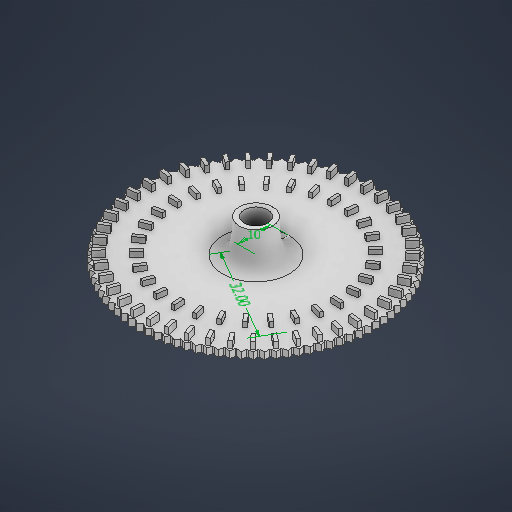
# Autodesk Inventor part: Диск v2
Saved by Autodesk Inventor 2026 (Build 300175000, 175)
## iProperties
Created: 2025-08-21
Part Number: Диск v2
Material: Типовые
Document SubType Name: Modeling
Designer: kvm13
Density: 1 g/cm^3
Appearance: По умолчанию
Author: kvm13
## iProperties of the stored document Диск v2_3DПЕЧАТЬ.ipt
Created: 2025-08-21
Part Number: Диск v2_3DПЕЧАТЬ
Material: Типовые
Document SubType Name: Modeling
Designer: kvm13
Density: 1 g/cm^3
Appearance: По умолчанию
Author: kvm13
Autodesk Inventor part; units mm, degrees
note: some values were not read from the file. Chosen so that the rebuilt part matches the saved one: pattern direction of "Круговой массив1".
ref_plane "YZ Plane" through (0, 0, 0) normal (1, 0, 0) x (0, 1, 0)
ref_plane "XZ Plane" through (0, 0, 0) normal (0, 1, 0) x (-1, 0, 0)
sketch "Эскиз1" plane through (0, 0, 0) normal (0, 1, 0) x (-1, 0, 0)
  circle A0 centre (0, 0) radius 35
  dimension "d0" = 70
  constraints: 1 centre point, 1 coincident
  measures "d0" diameter of A0
extrude "Выдавливание1" add sketch "Эскиз1" along normal blind 2
sketch "Эскиз2" plane through (0, 2, 0) normal (0, 1, 0) x (1, 0, 0)
  circle A0 centre (0, 0) radius 35 projected
  line L0 (0, 32) -> (-0.5, 32)
  line L1 (-0.5, 32) -> (-0.5, 34.9964)
  circle A1 centre (0, 0) radius 35 projected
  line L2 (0, 32) -> (0.5, 32)
  line L3 (0.5, 32) -> (0.5, 34.9964)
  dimension "d4" = 0.5
  constraints: 8 end point, 1 perpendicular, 3 other
  measures "d4" distance of L0.start L0.end
extrude "Выдавливание2" add sketch "Эскиз2" along normal blind 2 contours L3 L2 L0 L1 A0 picked at (-0.2222, 32.9999)
pattern_circular "Круговой массив1" count 45 over 360 about axis through (0, 0, 0) along (0, 1, 0) of "Выдавливание2"
sketch "Эскиз3" plane through (0, 2, 0) normal (0, 1, 0) x (1, 0, 0)
  line L0 (0.5, 32) -> (-0.5, 32) projected
  line L1 (-1.6712, 23.8986) -> (-1.1724, 23.9334)
  line L2 (-1.6712, 23.8986) -> (-2.1699, 23.8637)
  line L3 (-3.9584, 31.7582) -> (-4.3754, 34.7254) projected
  line L4 (-3.9584, 31.7582) -> (-0.5, 32)
  line L5 (-2.728, 31.8442) -> (-2.3792, 26.8564)
  line L6 (-2.3792, 26.8564) -> (-1.3816, 26.9261)
  line L7 (-1.3816, 26.9261) -> (-1.1724, 23.9334)
  line L8 (-2.3792, 26.8564) -> (-2.1699, 23.8637)
  point P0 (0, 0)
  point P1 (-1.4218, 23.916)
  dimension "d11" = 0.5
  dimension "d39" = 5
  dimension "d40" = 3
  constraints: 14 end point, 1 midpoint, 1 parallel
  measures "d11" distance of L1.start L1.end
  measures "d39" distance of L5.start L5.end
  measures "d40" distance of L5.end L2.end
extrude "Выдавливание3" add sketch "Эскиз3" along normal blind 1.5
sketch "Эскиз4" plane through (0, 0, 0) normal (0, -1, 0) x (1, 0, 0)
  line L0 (0, -35) -> (0, -36)
  line L1 (0, -36) -> (1.0147, -34.9853)
  line L2 (0, -36) -> (-1.0147, -34.9853)
  circle A0 centre (0, 0) radius 35
  dimension "d14" = 1
  dimension "d15" = 45
  constraints: 6 end point, 1 centre point, 1 coincident, 1 symmetric about line, 1 vertical
  measures "d14" distance of L0.start L0.end
  measures "d15" angle of L1 L0
extrude "Выдавливание4" add sketch "Эскиз4" against normal up to surface (2 mm away) contours A0 L1 L0 | L0 L2 A0
pattern_circular "Круговой массив2" count 90 over 360 about axis through (0, 0, 0) along (0, 1, 0) of "Выдавливание4"
pattern_circular "Круговой массив3" count 30 over 360 about axis through (0, 0, 0) along (0, 1, 0) of "Выдавливание3"
sketch "Эскиз5" plane through (0, 2, 0) normal (0, 1, 0) x (1, 0, 0)
  line L0 (0, 0) -> (0, 10)
  dimension "d24" = 10
  constraints: 2 end point, 1 vertical
  measures "d24" distance of L0.start L0.end
ref_plane "РабПлоскость1" through (0, 2, 0) normal (1, 0, 0) x (0, 0, -1)
sketch "Эскиз6" plane through (0, 2, 0) normal (1, 0, 0) x (0, 0, -1)
  line L0 (0, 0) -> (0, 10)
  line L1 (0, 0) -> (10, 0)
  line L2 (0, 0) -> (10, 0) projected
  line L3 (5, 10) -> (5, 2.9221) construction
  line L4 (5, 2.9221) -> (5.8227, 0) construction
  line L5 (5.8227, 0) -> (10, 0) construction
  spline S0 degree 3 poles (5, 10) (5, 2.9221) (5.8227, 0) (10, 0) knots 1 1 1 1 2 2 2 2
  line L6 (0, 10) -> (5, 10)
  point P0 (0, -2)
  dimension "d28" = 10
  dimension "d29" = 10
  dimension "d31" = 5
  constraints: 6 end point, 1 horizontal, 1 point on line, 1 vertical, 3 other
  measures "d28" distance of L0.start L1.end
  measures "d29" distance of L0.start L0.end
  measures "d31" distance of L0.end L3.start
revolve "Вращение1" add sketch "Эскиз6" angle 360 about axis through (0, 2, 0) along (0, 1, 0)
sketch "Эскиз7" plane through (0, 12, 0) normal (0, 1, 0) x (1, 0, 0)
  circle A0 centre (0, 0) radius 3.5
  point P0 (0, 0)
  dimension "d32" = 7
  constraints: 1 centre point, 1 coincident
  measures "d32" diameter of A0
extrude "Выдавливание5" cut sketch "Эскиз7" against normal blind 10
